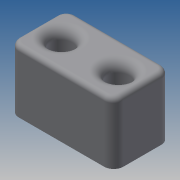
# Autodesk Inventor part: spacer
Saved by Autodesk Inventor 2014 (Build 180170000, 170)
## iProperties
Created: 2014-01-25
Part Number: spacer
Material: Generic
Document SubType Name: Modeling
Designer: Peele
Density: 1 g/cm^3
Appearance: Default
Author: Peele
Autodesk Inventor part; units mm, degrees
ref_plane "YZ Plane" through (0, 0, 0) normal (1, 0, 0) x (0, 1, 0)
ref_plane "XZ Plane" through (0, 0, 0) normal (0, 1, 0) x (-1, 0, 0)
ref_plane "XY Plane" through (0, 0, 0) normal (0, 0, 1) x (1, 0, 0)
sketch "Sketch1" plane through (0, 0, 0) normal (0, 0, 1) x (1, 0, 0)
  line L0 (-11, -6) -> (11, -6)
  line L1 (11, -6) -> (11, 6)
  line L2 (11, 6) -> (-11, 6)
  line L3 (-11, 6) -> (-11, -6)
  line L4 (-11, -6) -> (11, 6) construction
  line L5 (11, -6) -> (-11, 6) construction
  circle A0 centre (-6, 0) radius 2.3
  circle A1 centre (6, 0) radius 2.3
  line L6 (-6, 0) -> (0, 0) construction
  line L7 (0, 0) -> (6, 0) construction
  dimension "d0" = 12
  dimension "d1" = 4.6
  dimension "d2" = 12
  dimension "d3" = 5
  constraints: 16 end point, 3 equal length, 2 centre point, 2 midpoint, 2 perpendicular, 1 collinear, 1 equal radius, 1 horizontal
  measures "d0" distance of L7.end L6.start
  measures "d1" diameter of A0
  measures "d2" distance of L2.end L0.start
  measures "d3" distance from line of L6.start L3
extrude "Extrusion1" add sketch "Sketch1" along normal blind 13
fillet "Fillet1" radius 2 6 edges at (11, 6, 6.5) (11, -6, 6.5) (-11, 6, 6.5) (-11, -6, 6.5) (-8.3, 0, 13) (3.7, 0, 13)
fillet "Fillet2" radius 1 8 edges at (-10.4142, 5.4142, 13) (-11, 0, 13) (-10.4142, -5.4142, 13) (0, -6, 13) (10.4142, -5.4142, 13) (11, 0, 13) (10.4142, 5.4142, 13) (0, 6, 13)
body "Solid1"
